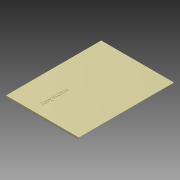
# Autodesk Inventor part: SidePanelwide
Saved by Autodesk Inventor 2015 (Build 190159000, 159)
## iProperties
Created: 2015-04-21
Part Number: SidePanelwide
Material: Nylon 6
Document SubType Name: Modeling
Designer: Akovo_000
Mass: 22.9058 g
Surface Area: 566.721 cm^2
Volume: 20.4516 cm^3
Density: 1.12 g/cm^3
Appearance: Nylon 6
Author: Akovo_000
Autodesk Inventor part; units mm, degrees
ref_plane "YZ Plane" through (0, 0, 0) normal (1, 0, 0) x (0, 1, 0)
ref_plane "XZ Plane" through (0, 0, 0) normal (0, 1, 0) x (-1, 0, 0)
ref_plane "XY Plane" through (0, 0, 0) normal (0, 0, 1) x (1, 0, 0)
sketch "PanelBody" plane through (0, 0, 0) normal (0, 0, 1) x (1, 0, 0)
  line L0 (-106.0995, 50.5777) -> (33.9005, 50.5777)
  line L1 (33.9005, 50.5777) -> (33.9005, -132.4223)
  line L2 (33.9005, -132.4223) -> (-106.0995, -132.4223)
  line L3 (-106.0995, -132.4223) -> (-106.0995, 50.5777)
  dimension "d1" = 140
  dimension "d2" = 183
  constraints: 8 end point, 2 parallel, 1 horizontal, 1 perpendicular
  measures "d1" distance of L1.end L2.end
  measures "d2" distance of L0.end L1.end
extrude "PanelFace" add sketch "PanelBody" along normal blind 2
sketch "SideHooks" plane through (-106.0995, -132.4223, 0) normal (-1, 0, 0) x (0, 0, 1)
  line L0 (0, 183) -> (-1.9, 183)
  line L1 (-1.9, 183) -> (-1.9, 181.1)
  line L2 (-1.9, 181.1) -> (0, 181.1)
  line L3 (0, 181.1) -> (0, 183)
  line L4 (0, 0) -> (-1.9, 0)
  line L5 (-1.9, 0) -> (-1.9, 1.9)
  line L6 (-1.9, 1.9) -> (0, 1.9)
  line L7 (0, 1.9) -> (0, 0)
  line L8 (0, 0) -> (2, 0) projected
  point P0 (0, 132.4223)
  dimension "d33" = 1.9
  constraints: 16 end point, 4 parallel, 3 equal length, 2 horizontal, 2 perpendicular
  measures "d33" distance of L5.end L6.end
extrude "Corners" add sketch "SideHooks" against normal blind 140
sketch "Sketch3" plane through (33.9005, 50.5777, -1.9) normal (0, 0, -1) x (-1, 0, 0)
  line L0 (0, -183) -> (140, -183) construction
  line L1 (140, -183) -> (140, 0) construction
  line L2 (140, 0) -> (0, 0) construction
  line L3 (0, 0) -> (0, -183) construction
  line L4 (137.5, -180.5) -> (133.9364, -180.5) construction
  line L5 (72.5, -165.5) -> (72.5, -107.1428)
  line L6 (137.5, -109) -> (137.5, -171.0951)
  line L7 (137.5, -2.5) -> (133.9364, -2.5) construction
  line L8 (72.5, -17.5) -> (72.5, -75.8572)
  line L9 (137.5, -74) -> (137.5, -11.9049)
  line L10 (2.5, -2.5) -> (6.0636, -2.5) construction
  line L11 (67.5, -17.5) -> (67.5, -75.8572)
  line L12 (2.5, -74) -> (2.5, -11.9049)
  line L13 (2.5, -180.5) -> (6.0636, -180.5) construction
  line L14 (67.5, -165.5) -> (67.5, -107.1428)
  line L15 (2.5, -109) -> (2.5, -171.0951)
  line L16 (72.5, -2.5) -> (67.5, -2.5) construction
  line L17 (2.5, -89) -> (2.5, -94) construction
  line L18 (67.5, -180.5) -> (72.5, -180.5) construction
  line L19 (137.5, -89) -> (137.5, -94) construction
  line L20 (133.9197, -10.679) -> (75.6664, -85.7741)
  line L21 (76.0803, -77.0831) -> (131.434, -5.7259)
  line L22 (63.9197, -77.0831) -> (8.566, -5.7259)
  line L23 (64.3336, -85.7741) -> (6.0803, -10.679)
  line L24 (10.1463, -2.5) -> (52.5, -2.5)
  line L25 (2.5, -6.0636) -> (2.5, -2.5) construction
  line L26 (77.2467, -89) -> (122.5, -89)
  line L27 (137.5, -6.0636) -> (137.5, -2.5) construction
  line L28 (129.8537, -2.5) -> (87.5, -2.5)
  line L29 (62.7533, -89) -> (17.5, -89)
  line L30 (133.9197, -172.321) -> (75.6664, -97.2259)
  line L31 (76.0803, -105.9169) -> (131.434, -177.2741)
  line L32 (63.9197, -105.9169) -> (8.566, -177.2741)
  line L33 (6.0803, -172.321) -> (64.3336, -97.2259)
  line L34 (77.2467, -94) -> (122.5, -94)
  line L35 (62.7533, -94) -> (17.5, -94)
  line L36 (2.5, -176.9364) -> (2.5, -180.5) construction
  line L37 (10.1463, -180.5) -> (52.5, -180.5)
  line L38 (129.8537, -180.5) -> (87.5, -180.5)
  line L39 (137.5, -176.9364) -> (137.5, -180.5) construction
  line L40 (140, -183) -> (0, -183) projected
  line L41 (140, 0) -> (0, 0) projected
  line L42 (0, -1.9) -> (0, -181.1) projected
  line L43 (140, 0) -> (140, -1.9) projected
  arc A0 (52.5, -180.5) -> (67.5, -165.5) centre (52.5, -165.5) ccw
  arc A1 (72.5, -165.5) -> (87.5, -180.5) centre (87.5, -165.5) ccw
  arc A2 (87.5, -2.5) -> (72.5, -17.5) centre (87.5, -17.5) ccw
  arc A3 (67.5, -17.5) -> (52.5, -2.5) centre (52.5, -17.5) ccw
  arc A4 (122.5, -89) -> (137.5, -74) centre (122.5, -74) ccw
  arc A5 (137.5, -109) -> (122.5, -94) centre (122.5, -109) ccw
  arc A6 (17.5, -94) -> (2.5, -109) centre (17.5, -109) ccw
  arc A7 (2.5, -74) -> (17.5, -89) centre (17.5, -74) ccw
  arc A8 (8.566, -177.2741) -> (10.1463, -180.5) centre (10.1463, -178.5) ccw
  arc A9 (2.5, -171.0951) -> (6.0803, -172.321) centre (4.5, -171.0951) ccw
  arc A10 (64.3336, -97.2259) -> (62.7533, -94) centre (62.7533, -96) ccw
  arc A11 (62.7533, -89) -> (64.3336, -85.7741) centre (62.7533, -87) ccw
  arc A12 (72.5, -75.8572) -> (76.0803, -77.0831) centre (74.5, -75.8572) ccw
  arc A13 (63.9197, -77.0831) -> (67.5, -75.8572) centre (65.5, -75.8572) ccw
  arc A14 (131.434, -5.7259) -> (129.8537, -2.5) centre (129.8537, -4.5) ccw
  arc A15 (10.1463, -2.5) -> (8.566, -5.7259) centre (10.1463, -4.5) ccw
  arc A16 (6.0803, -10.679) -> (2.5, -11.9049) centre (4.5, -11.9049) ccw
  arc A17 (75.6664, -85.7741) -> (77.2467, -89) centre (77.2467, -87) ccw
  arc A18 (77.2467, -94) -> (75.6664, -97.2259) centre (77.2467, -96) ccw
  arc A19 (133.9197, -172.321) -> (137.5, -171.0951) centre (135.5, -171.0951) ccw
  arc A20 (129.8537, -180.5) -> (131.434, -177.2741) centre (129.8537, -178.5) ccw
  arc A21 (76.0803, -105.9169) -> (72.5, -107.1428) centre (74.5, -107.1428) ccw
  arc A22 (67.5, -107.1428) -> (63.9197, -105.9169) centre (65.5, -107.1428) ccw
  arc A23 (137.5, -11.9049) -> (133.9197, -10.679) centre (135.5, -11.9049) ccw
  point P0 (73.164, -89)
  point P1 (72.5, -81.6985)
  point P2 (67.5, -81.6985)
  point P3 (66.836, -89)
  point P4 (73.164, -94)
  point P5 (72.5, -101.3015)
  point P6 (67.5, -101.3015)
  point P7 (66.836, -94)
  dimension "d16" = 2.5
  dimension "d25" = 5
  dimension "d26" = 2.5
  dimension "d27" = 2.5
  dimension "d28" = 2.5
  dimension "d34" = 0
  dimension "d36" = 0
  dimension "d37" = 0
  dimension "d38" = 0
  dimension "d46" = 5
  dimension "d47" = 5
  dimension "d48" = 15
  dimension "d49" = 2
  constraints: 80 end point, 49 point on line, 48 point on circle, 48 tangent, 24 centre point, 22 equal radius, 15 equal length, 10 horizontal, 8 parallel, 7 collinear, 6 vertical, 3 perpendicular
  measures "d16" distance between parallel lines of L10 L2
  measures "d25" distance of L17.start L17.end
  measures "d26" horizontal distance of L0.start L13.start
  measures "d27" horizontal distance of L1.end L7.start
  measures "d28" horizontal distance of L0.end L4.start
  measures "d34" distance from line of L40 L0.start
  measures "d36" distance between parallel lines of L41 L2
  measures "d37" distance between parallel lines of L42 L3
  measures "d38" distance between parallel lines of L43 L1
  measures "d46" distance of L16.start L16.end
  measures "d47" distance between parallel lines of L22 L23
  measures "d48" radius of A0
  measures "d49" radius of A8
extrude "ReinforcementBars" cut sketch "Sketch3" against normal blind 3.5
sketch "Sketch4" plane through (0, 0, 2) normal (0, 0, 1) x (1, 0, 0)
  line L0 (-62.4757, -113.2868) -> (-62.4757, -58.6034) construction
  line L1 (-62.4757, -58.6034) -> (1.9126, -58.6034) construction
  line L2 (1.9126, -58.6034) -> (1.9126, -113.2868) construction
  line L3 (1.9126, -113.2868) -> (-62.4757, -113.2868) construction
  line L4 (-54.4757, -113.3193) -> (-62.4757, -110.6158)
  line L5 (-62.4757, -110.6158) -> (-62.4757, -108.4246)
  line L6 (-62.4757, -108.4246) -> (-54.4757, -105.7212)
  line L7 (-54.4757, -105.7212) -> (-54.4757, -107.7893)
  line L8 (-54.4757, -107.7893) -> (-56.1094, -108.2885)
  line L9 (-56.1094, -108.2885) -> (-56.1094, -110.8039)
  line L10 (-56.1094, -110.8039) -> (-54.4757, -111.3095)
  line L11 (-54.4757, -111.3095) -> (-54.4757, -113.3193)
  line L12 (-57.5616, -108.7293) -> (-60.2066, -109.5462)
  line L13 (-60.2066, -109.5462) -> (-57.5616, -110.3695)
  line L14 (-57.5616, -110.3695) -> (-57.5616, -108.7293)
  line L15 (-54.4757, -99.3873) -> (-54.4757, -101.2804)
  line L16 (-54.4757, -101.2804) -> (-57.4643, -101.2804)
  spline S0 degree 2 poles (-57.4643, -101.2804) (-57.8339, -101.2804) (-58.56, -101.3387) (-58.7285, -101.4165) knots 0 0 0 1 2 2 2
  spline S1 degree 2 poles (-58.7285, -101.4165) (-58.936, -101.5137) (-59.111, -101.8768) (-59.111, -102.188) knots 0 0 0 1 2 2 2
  spline S2 degree 2 poles (-59.111, -102.188) (-59.111, -102.4149) (-58.936, -102.8881) (-58.748, -103.1539) knots 0 0 0 1 2 2 2
  line L17 (-58.748, -103.1539) -> (-54.4757, -103.1539)
  line L18 (-54.4757, -103.1539) -> (-54.4757, -105.034)
  line L19 (-54.4757, -105.034) -> (-60.5113, -105.034)
  line L20 (-60.5113, -105.034) -> (-60.5113, -103.1539)
  line L21 (-60.5113, -103.1539) -> (-59.8436, -103.1539)
  spline S3 degree 2 poles (-59.8436, -103.1539) (-60.2326, -102.6936) (-60.6734, -101.8184) (-60.6734, -101.2868) knots 0 0 0 1 2 2 2
  spline S4 degree 2 poles (-60.6734, -101.2868) (-60.6734, -100.3663) (-59.5065, -99.3873) (-58.4044, -99.3873) knots 0 0 0 1 2 2 2
  line L22 (-58.4044, -99.3873) -> (-54.4757, -99.3873)
  line L23 (-60.5113, -92.3663) -> (-52.265, -95.4068)
  line L24 (-52.265, -95.4068) -> (-52.265, -97.4295)
  line L25 (-52.265, -97.4295) -> (-54.6248, -96.5154)
  line L26 (-54.6248, -96.5154) -> (-60.5113, -98.7261)
  line L27 (-60.5113, -98.7261) -> (-60.5113, -96.7552)
  line L28 (-60.5113, -96.7552) -> (-56.7253, -95.4846)
  line L29 (-56.7253, -95.4846) -> (-60.5113, -94.2982)
  line L30 (-60.5113, -94.2982) -> (-60.5113, -92.3663)
  line L31 (-60.5113, -82.6677) -> (-54.4757, -84.4311)
  line L32 (-54.4757, -84.4311) -> (-54.4757, -86.4278)
  line L33 (-54.4757, -86.4278) -> (-58.3784, -87.491)
  line L34 (-58.3784, -87.491) -> (-54.4757, -88.5543)
  line L35 (-54.4757, -88.5543) -> (-54.4757, -90.551)
  line L36 (-54.4757, -90.551) -> (-60.5113, -92.3014)
  line L37 (-60.5113, -92.3014) -> (-60.5113, -90.3241)
  line L38 (-60.5113, -90.3241) -> (-56.5178, -89.397)
  line L39 (-56.5178, -89.397) -> (-60.5113, -88.256)
  line L40 (-60.5113, -88.256) -> (-60.5113, -86.5899)
  line L41 (-60.5113, -86.5899) -> (-56.5178, -85.5137)
  line L42 (-56.5178, -85.5137) -> (-60.5113, -84.5996)
  line L43 (-60.5113, -84.5996) -> (-60.5113, -82.6677)
  spline S5 degree 2 poles (-55.1175, -78.5445) (-54.9554, -78.739) (-54.6961, -79.0437) (-54.5665, -79.303) knots 0 0 0 1 2 2 2
  spline S6 degree 2 poles (-54.5665, -79.303) (-54.4433, -79.5559) (-54.3136, -80.0356) (-54.3136, -80.4635) knots 0 0 0 1 2 2 2
  spline S7 degree 2 poles (-54.3136, -80.4635) (-54.3136, -81.2674) (-55.3898, -82.3241) (-56.2066, -82.3241) knots 0 0 0 1 2 2 2
  spline S8 degree 2 poles (-56.2066, -82.3241) (-56.8744, -82.3241) (-57.7042, -81.786) (-57.9441, -81.2804) knots 0 0 0 1 2 2 2
  spline S9 degree 2 poles (-57.9441, -81.2804) (-58.1904, -80.7682) (-58.3849, -79.3484) (-58.4368, -78.5316) knots 0 0 0 1 2 2 2
  line L44 (-58.4368, -78.5316) -> (-58.4692, -78.5316)
  spline S10 degree 2 poles (-58.4692, -78.5316) (-58.9684, -78.5316) (-59.3509, -79.2706) (-59.3509, -80.0097) knots 0 0 0 1 2 2 2
  spline S11 degree 2 poles (-59.3509, -80.0097) (-59.3509, -80.3403) (-59.111, -81.235) (-58.923, -81.6564) knots 0 0 0 1 2 2 2
  line L45 (-58.923, -81.6564) -> (-58.923, -81.8184)
  line L46 (-58.923, -81.8184) -> (-60.3817, -81.8184)
  spline S12 degree 2 poles (-60.3817, -81.8184) (-60.4595, -81.5397) (-60.6799, -80.2949) (-60.6799, -79.6596) knots 0 0 0 1 2 2 2
  spline S13 degree 2 poles (-60.6799, -79.6596) (-60.6799, -78.1037) (-59.6426, -76.6774) (-58.5794, -76.6774) knots 0 0 0 1 2 2 2
  line L47 (-58.5794, -76.6774) -> (-54.4757, -76.6774)
  line L48 (-54.4757, -76.6774) -> (-54.4757, -78.5445)
  line L49 (-54.4757, -78.5445) -> (-55.1175, -78.5445)
  line L50 (-56.0511, -78.5445) -> (-57.3023, -78.5445)
  spline S14 degree 2 poles (-57.3023, -78.5445) (-57.2569, -79.0243) (-57.1856, -79.6142) (-57.0818, -79.8995) knots 0 0 0 1 2 2 2
  spline S15 degree 2 poles (-57.0818, -79.8995) (-56.9976, -80.1523) (-56.6475, -80.4246) (-56.3622, -80.4246) knots 0 0 0 1 2 2 2
  spline S16 degree 2 poles (-56.3622, -80.4246) (-55.9408, -80.4246) (-55.6232, -79.9643) (-55.6232, -79.517) knots 0 0 0 1 2 2 2
  spline S17 degree 2 poles (-55.6232, -79.517) (-55.6232, -79.2706) (-55.8501, -78.752) (-56.0511, -78.5445) knots 0 0 0 1 2 2 2
  line L51 (-60.5113, -69.6369) -> (-54.4757, -71.8022)
  line L52 (-54.4757, -71.8022) -> (-54.4757, -73.8573)
  line L53 (-54.4757, -73.8573) -> (-60.5113, -76.0032)
  line L54 (-60.5113, -76.0032) -> (-60.5113, -74.0259)
  line L55 (-60.5113, -74.0259) -> (-56.5243, -72.7941)
  line L56 (-56.5243, -72.7941) -> (-60.5113, -71.5753)
  line L57 (-60.5113, -71.5753) -> (-60.5113, -69.6369)
  spline S18 degree 2 poles (-54.3136, -65.8249) (-54.3136, -67.5364) (-55.9473, -69.3581) (-57.4579, -69.3581) knots 0 0 0 1 2 2 2
  spline S19 degree 2 poles (-57.4579, -69.3581) (-58.936, -69.3581) (-60.6994, -67.6596) (-60.6994, -66.1296) knots 0 0 0 1 2 2 2
  spline S20 degree 2 poles (-60.6994, -66.1296) (-60.6994, -64.7487) (-59.2018, -63.3484) (-57.8144, -63.3484) knots 0 0 0 1 2 2 2
  line L58 (-57.8144, -63.3484) -> (-57.1337, -63.3484)
  line L59 (-57.1337, -63.3484) -> (-57.1337, -67.4781)
  spline S21 degree 2 poles (-57.1337, -67.4781) (-56.7123, -67.4522) (-56.1548, -67.1475) (-55.9862, -66.9011) knots 0 0 0 1 2 2 2
  spline S22 degree 2 poles (-55.9862, -66.9011) (-55.8177, -66.6612) (-55.675, -66.0129) (-55.675, -65.6304) knots 0 0 0 1 2 2 2
  spline S23 degree 2 poles (-55.675, -65.6304) (-55.675, -65.3063) (-55.8177, -64.671) (-55.9408, -64.4051) knots 0 0 0 1 2 2 2
  spline S24 degree 2 poles (-55.9408, -64.4051) (-56.0381, -64.1718) (-56.278, -63.7828) (-56.3687, -63.6596) knots 0 0 0 1 2 2 2
  line L60 (-56.3687, -63.6596) -> (-56.3687, -63.4586)
  line L61 (-56.3687, -63.4586) -> (-54.8128, -63.4586)
  spline S25 degree 2 poles (-54.8128, -63.4586) (-54.722, -63.692) (-54.5665, -64.068) (-54.4887, -64.4051) knots 0 0 0 1 2 2 2
  spline S26 degree 2 poles (-54.4887, -64.4051) (-54.4044, -64.7098) (-54.3136, -65.3581) (-54.3136, -65.8249) knots 0 0 0 1 2 2 2
  spline S27 degree 2 poles (-58.2682, -65.2026) (-58.8647, -65.2155) (-59.4935, -65.7406) (-59.4935, -66.2787) knots 0 0 0 1 2 2 2
  spline S28 degree 2 poles (-59.4935, -66.2787) (-59.4935, -66.8298) (-58.8323, -67.4522) (-58.2682, -67.4846) knots 0 0 0 1 2 2 2
  line L62 (-58.2682, -67.4846) -> (-58.2682, -65.2026)
  point P0 (0, 0)
  constraints: 2 other
extrude "Extrusion4" add sketch "Sketch4" along normal blind 0.5
body "Solid1"
